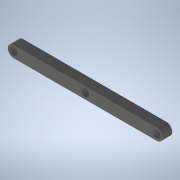
# Autodesk Inventor part: Lever
Saved by Autodesk Inventor 2022 (Build 260153000, 153)
## iProperties
Created: 2021-12-04
Part Number: Lever
Material: Generic
Document SubType Name: Modeling
Designer: LEGION SMIT
Density: 1 g/cm^3
Appearance: Generic
Author: LEGION SMIT
Autodesk Inventor part; units mm, degrees
ref_plane "YZ Plane" through (0, 0, 0) normal (1, 0, 0) x (0, 1, 0)
ref_plane "XZ Plane" through (0, 0, 0) normal (0, 1, 0) x (-1, 0, 0)
sketch "Sketch1" plane through (0, 0, 0) normal (0, 0, 1) x (1, 0, 0)
  circle A0 centre (0, 0) radius 4
  circle A1 centre (0, 0) radius 5
  line L0 (-90, -6) -> (90, -6)
  line L1 (90, -6) -> (90, 6)
  line L2 (90, 6) -> (-90, 6)
  line L3 (-90, 6) -> (-90, -6)
  line L4 (-90, -6) -> (90, 6) construction
  line L5 (90, -6) -> (-90, 6) construction
  point P0 (0, -5)
  point P1 (0, 5)
  point P2 (0, 0)
  point P3 (0, 0)
  dimension "d11" = 180
  dimension "d14" = 12
  constraints: 12 end point, 3 midpoint, 2 centre point, 2 coincident, 2 parallel, 1 horizontal, 1 perpendicular
  measures "d11" distance of L2.end L1.end
  measures "d14" distance between parallel lines of L0 L2
ref_plane "Work Plane1" through (0, 0, 5) normal (0, 0, 1) x (1, 0, 0)
extrude "Extrusion3" add sketch "Sketch1" along normal mid plane 10 contours A0 | A1 | L3 L2 L1 L0
extrude "Extrusion4" cut sketch "Sketch1" along normal mid plane 10 contours A0
fillet "Fillet3" radius 6 4 edges at (-90, -6, 0) (-90, 6, 0) (90, 6, 0) (90, -6, 0)
sketch "Sketch4" plane through (0, 0, 5) normal (0, 0, 1) x (1, 0, 0)
  circle A0 centre (0, 0) radius 4 projected
  line L0 (0, 0) -> (-80, 0)
  circle A1 centre (-80, 0) radius 4
  circle A2 centre (-80, 0) radius 6
  line L1 (-84, 6) -> (84, 6) projected
  point P0 (0, 0)
  dimension "d22" = 80
  dimension "d23" = 8
  constraints: 2 centre point, 2 coincident, 2 end point, 1 horizontal, 1 tangent
  measures "d22" distance of L0.start L0.end
  measures "d23" diameter of A1
extrude "Extrusion6" cut sketch "Sketch4" against normal blind 10 contours A1
mirror "Mirror2" about plane through (0, 0, 0) normal (1, 0, 0) of "Extrusion6"
body "Solid1"
